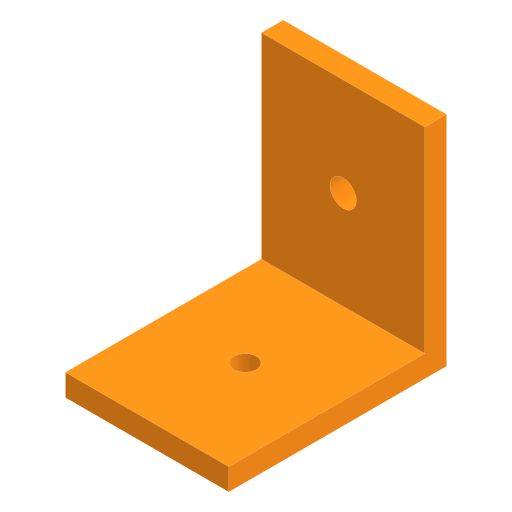
# Autodesk Inventor part: 30x30_angle
Saved by Autodesk Inventor 2023.1 (Build 271208000, 208)
## iProperties
Created: 2023-07-01
Part Number: 30x30_angle
Material: Stainless Steel
Document SubType Name: Modeling
Designer: queezz
Density: 8 g/cm^3
Appearance: Orange
Mass: 71.9181 g
Surface Area: 54.5699 cm^2
Volume: 8.98977 cm^3
Author: queezz
Autodesk Inventor part; units mm, degrees
ref_plane "YZ Plane" through (0, 0, 0) normal (1, 0, 0) x (0, 1, 0)
ref_plane "XZ Plane" through (0, 0, 0) normal (0, 1, 0) x (-1, 0, 0)
ref_plane "XY Plane" through (0, 0, 0) normal (0, 0, 1) x (1, 0, 0)
sketch "Sketch1" plane through (0, 0, 0) normal (1, 0, 0) x (0, 1, 0)
  line L0 (0, 0) -> (0, 40)
  line L1 (0, 40) -> (4, 40)
  line L2 (4, 40) -> (4, 4)
  line L3 (4, 4) -> (40, 4)
  line L4 (40, 4) -> (40, 0)
  line L5 (40, 0) -> (0, 0)
  dimension "d0" = 40
  dimension "d1" = 4
  constraints: 12 end point, 7 perpendicular, 1 vertical
  measures "d0" distance of L4.end L0.start
  measures "d1" distance of L3.end L4.end
extrude "Extrusion1" add sketch "Sketch1" along normal mid plane 30
sketch "Sketch4" plane through (-15, 4, 4) normal (0, 0, 1) x (1, 0, 0)
  circle A0 centre (15, 18) radius 2.44
  line L0 (30, 36) -> (30, 0) projected
  line L1 (0, 36) -> (30, 36) projected
  point P0 (15, -4)
  point P1 (30, 18)
  point P2 (15, 36)
  constraints: 2 midpoint, 1 centre point, 1 horizontal alignment, 1 vertical alignment
extrude "Extrusion3" cut sketch "Sketch4" against normal blind 10
sketch "Sketch5" plane through (-15, 4, 40) normal (0, 1, 0) x (1, 0, 0)
  line L0 (0, 0) -> (30, 0) projected
  line L1 (30, 36) -> (30, 0) projected
  line L2 (0, 36) -> (30, 36) projected
  line L3 (0, 0) -> (0, 36) projected
  circle A0 centre (15, 18) radius 2.1
  point P0 (15, 40)
  point P1 (30, 18)
  point P2 (15, 0)
  dimension "d9" = 4.2
  constraints: 2 midpoint, 1 centre point, 1 horizontal alignment, 1 vertical alignment
  measures "d9" diameter of A0
extrude "Extrusion4" cut sketch "Sketch5" against normal through all contours A0
body "Solid1"
